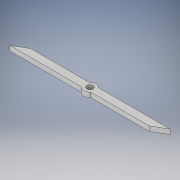
# Autodesk Inventor part: Propeller
Saved by Autodesk Inventor 2019 (Build 230136000, 136)
## iProperties
Created: 2019-06-19
Part Number: Propeller
Material: Generic
Document SubType Name: Modeling
Designer: abdel
Density: 1 g/cm^3
Appearance: Default
Author: abdel
Autodesk Inventor part; units mm, degrees
ref_plane "YZ Plane" through (0, 0, 0) normal (1, 0, 0) x (0, 1, 0)
ref_plane "XZ Plane" through (0, 0, 0) normal (0, 1, 0) x (-1, 0, 0)
ref_plane "XY Plane" through (0, 0, 0) normal (0, 0, 1) x (1, 0, 0)
sketch "Sketch1" plane through (0, 0, 0) normal (0, 1, 0) x (-1, 0, 0)
  circle A0 centre (0, 0) radius 4.2386
  circle A1 centre (0, 0) radius 8.0486
  line L0 (-101.6, -5.08) -> (-84.0024, 5.08)
  line L1 (-101.6, -5.08) -> (-81.28, -5.08) construction
  line L2 (101.6, 5.08) -> (84.0024, -5.08)
  line L3 (84.0024, -5.08) -> (6.2429, -5.08)
  line L4 (-6.2429, -5.08) -> (-101.6, -5.08)
  line L5 (101.6, 5.08) -> (6.2429, 5.08)
  line L6 (-6.2429, 5.08) -> (-84.0024, 5.08)
  dimension "d0" = 8.4772
  dimension "d2" = 3.81
  dimension "d8" = 30
  constraints: 14 end point, 4 point on circle, 2 centre point, 1 coincident, 1 equal length, 1 horizontal
  measures "d0" diameter of A0
  measures "d2" radial gap between concentric circles of A0 A1
  measures "d8" angle of L1 L0
extrude "Extrusion1" add sketch "Sketch1" along normal blind 6.35
body "Solid1"
